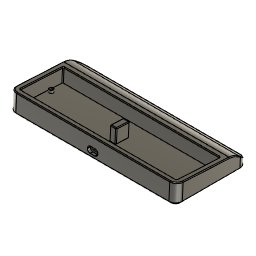
SK-Tsuru (Autodesk Fusion 360 design; units mm, degrees)
Autodesk Fusion 360 part; units mm, degrees
sketch "Base Plane Sketch" plane through (0, 0, 0) normal (0, 0, 1) x (1, 0, 0)
  line L0 (45.9345, 28.7794) -> (255.4845, 28.7794) construction
  line L1 (255.4845, 28.7794) -> (255.4845, 85.9294) construction
  line L2 (255.4845, 85.9294) -> (45.9345, 85.9294) construction
  line L3 (45.9345, 85.9294) -> (45.9345, 28.7794) construction
  line L4 (255.9845, 86.4294) -> (45.4345, 86.4294)
  line L5 (45.4345, 86.4294) -> (45.4345, 28.2794)
  line L6 (45.4345, 28.2794) -> (255.9845, 28.2794)
  line L7 (255.9845, 28.2794) -> (255.9845, 86.4294)
  line L8 (262.8595, 93.3044) -> (38.5595, 93.3044)
  line L9 (38.5595, 93.3044) -> (38.5595, 21.4044)
  line L10 (38.5595, 21.4044) -> (262.8595, 21.4044)
  line L11 (262.8595, 21.4044) -> (262.8595, 93.3044)
  dimension "d180" = 209.55
  dimension "d181" = 57.15
  dimension "d182" = 0.5
  dimension "d183" = 7.375
  constraint horizontal L0
  constraint vertical L1
  constraint horizontal L2
  constraint vertical L3
  measures "d180" distance of L0.start L0.end
  measures "d181" distance of L0.start L2.end
extrude "Extrude19" add sketch "Base Plane Sketch" along normal blind 21.06
extrude "Extrude20" add sketch "Base Plane Sketch" along normal blind 3 contours L4 L5 L6 L7
sketch "Side Plane Sketch" plane through (262.8595, 0, 0) normal (1, 0, 0) x (0, 1, 0)
  line L0 (21.4044, 0) -> (93.3044, 0)
  line L1 (93.3044, 0) -> (93.3044, 21.06)
  line L2 (93.3044, 21.06) -> (21.4044, 21.06)
  line L3 (21.4044, 21.06) -> (21.4044, 0)
  line L4 (93.3044, 21.06) -> (99.8544, 21.06)
  line L5 (99.8544, 21.06) -> (117.0144, 10.0011)
  line L6 (99.8544, 21.06) -> (124.9018, 21.06) construction
  line L7 (93.3044, 0) -> (117.0144, 0)
  line L8 (117.0144, 0) -> (117.0144, 10.0011)
  dimension "d188" = 6.55
  dimension "d189" = 32.8
  dimension "d190" = 23.71
  constraint coincident L1.end L2.start
  constraint perpendicular L1 L4
  constraint horizontal L6
  constraint coincident L0.end L1.start
  constraint perpendicular L1 L7
  constraint perpendicular L7 L8
  measures "d188" distance of L1.end L4.end
  measures "d189" angle of L5 L6
  measures "d190" distance of L0.end L7.end
extrude "Extrude21" add sketch "Side Plane Sketch" against normal up to surface (224.3 mm away) contours L1 L4 L5 L7 L8
sketch "USB C Hole Internal Sketch" plane through (0, 28.2794, 0) normal (0, 1, 0) x (-1, 0, 0)
  line L0 (-255.9845, 3) -> (-45.4345, 3)
  line L1 (-45.4345, 3) -> (-45.4345, 21.06)
  line L2 (-45.4345, 21.06) -> (-255.9845, 21.06)
  line L3 (-255.9845, 21.06) -> (-255.9845, 3)
  line L4 (-255.4845, 21.06) -> (-255.4845, 3) construction
  line L5 (-255.4845, 3) -> (-150.7095, 3) construction
  line L6 (-150.7095, 3) -> (-150.7095, 4.83) construction
  line L7 (-145.9845, 6.66) -> (-155.4345, 6.66)
  line L8 (-155.4345, 6.66) -> (-155.4345, 3)
  line L9 (-155.4345, 3) -> (-145.9845, 3)
  line L10 (-145.9845, 3) -> (-145.9845, 6.66)
  line L11 (-145.9845, 6.66) -> (-155.4345, 3) construction
  line L12 (-155.4345, 6.66) -> (-145.9845, 3) construction
  point P0 (-150.7095, 4.83)
  dimension "d197" = -0.5
  dimension "d198" = 104.775
  dimension "d199" = 1.83
  dimension "d200" = 9.45
  dimension "d201" = 3.66
  constraint perpendicular L4 L5
  constraint perpendicular L5 L6
  constraint horizontal L7
  constraint perpendicular L7 L8
  constraint parallel L7 L9
  constraint parallel L8 L10
  constraint coincident L11 P0
  constraint coincident L12 P0
  constraint coincident P0 L6.end
  measures "d198" distance of L4.end L5.end
  measures "d199" distance of L5.end P0
  measures "d200" distance of L8.end L9.end
  measures "d201" distance of L7.end L8.end
extrude "Extrude22" cut sketch "USB C Hole Internal Sketch" against normal blind 15 contours L0 L7 L8 L9 L10
sketch "USB C Hole External Sketch" plane through (0, 21.4044, 0) normal (0, -1, 0) x (1, 0, 0)
  line L0 (145.9845, 6.66) -> (155.4345, 6.66)
  line L1 (155.4345, 6.66) -> (155.4345, 3)
  line L2 (155.4345, 3) -> (145.9845, 3)
  line L3 (145.9845, 3) -> (145.9845, 6.66)
  line L4 (38.5595, 0) -> (262.8595, 0)
  line L5 (262.8595, 0) -> (262.8595, 21.06)
  line L6 (262.8595, 21.06) -> (38.5595, 21.06)
  line L7 (38.5595, 21.06) -> (38.5595, 0)
  line L8 (145.9845, 3) -> (155.4345, 6.66) construction
  line L9 (155.4345, 3) -> (145.9845, 6.66) construction
  line L10 (157.6845, 8.91) -> (143.7345, 8.91)
  line L11 (143.7345, 8.91) -> (143.7345, 0.75)
  line L12 (143.7345, 0.75) -> (157.6845, 0.75)
  line L13 (157.6845, 0.75) -> (157.6845, 8.91)
  line L14 (157.6845, 8.91) -> (143.7345, 0.75) construction
  line L15 (143.7345, 8.91) -> (157.6845, 0.75) construction
  point P0 (150.7095, 4.83)
  dimension "d204" = 13.95
  dimension "d205" = 8.16
  constraint coincident L2.end L3.start
  constraint coincident L0.end L1.start
  constraint coincident L1.end L2.start
  constraint coincident L0.start L3.end
  constraint horizontal L10
  constraint perpendicular L10 L11
  constraint parallel L10 L12
  constraint parallel L11 L13
  constraint coincident L14 P0
  constraint coincident L15 P0
  constraint midpoint L8 P0
  measures "d204" distance of L11.end L12.end
  measures "d205" distance of L10.end L11.end
extrude "Extrude23" cut sketch "USB C Hole External Sketch" against normal blind 3.875 contours L10 L11 L12 L13
fillet "Fillet8" radius 1.55 4 edges at (145.9845, 26.7794, 3) (145.9845, 26.7794, 6.66) (155.4345, 26.7794, 3) (155.4345, 26.7794, 6.66)
fillet "Fillet9" radius 3.8 4 edges at (143.7345, 23.3419, 8.91) (157.6845, 23.3419, 8.91) (157.6845, 23.3419, 0.75) (143.7345, 23.3419, 0.75)
sketch "Screw Post and Center Blocker Sketch" plane through (0, 0, 3) normal (0, 0, 1) x (-1, 0, 0)
  line L0 (-153.8845, -25.2794) -> (-153.8845, -28.2794)
  line L1 (-153.8845, -28.2794) -> (-255.9845, -28.2794)
  line L2 (-255.9845, -28.2794) -> (-255.9845, -86.4294)
  line L3 (-255.9845, -86.4294) -> (-45.4345, -86.4294)
  line L4 (-45.4345, -86.4294) -> (-45.4345, -28.2794)
  line L5 (-45.4345, -28.2794) -> (-147.5345, -28.2794)
  line L6 (-147.5345, -28.2794) -> (-147.5345, -25.2794)
  line L7 (-147.5345, -25.2794) -> (-153.8845, -25.2794)
  line L8 (-45.9345, -28.7794) -> (-148.0345, -28.7794) construction
  line L9 (-148.0345, -28.7794) -> (-148.0345, -25.7794) construction
  line L10 (-148.0345, -25.7794) -> (-153.3845, -25.7794) construction
  line L11 (-153.3845, -25.7794) -> (-153.3845, -28.7794) construction
  line L12 (-153.3845, -28.7794) -> (-255.4845, -28.7794) construction
  line L13 (-255.4845, -28.7794) -> (-255.4845, -85.9294) construction
  line L14 (-255.4845, -85.9294) -> (-45.9345, -85.9294) construction
  line L15 (-45.9345, -85.9294) -> (-45.9345, -28.7794) construction
  circle A0 centre (-229.2905, -33.8394) radius 2.75
  circle A1 centre (-251.9125, -66.8794) radius 2.75
  circle A2 centre (-72.1285, -33.8394) radius 2.75
  circle A3 centre (-49.5065, -66.8794) radius 2.75
  line L16 (-255.4845, -28.7794) -> (-45.9345, -85.9294) construction
  line L17 (-45.9345, -28.7794) -> (-255.4845, -85.9294) construction
  line L18 (-145.947, -47.8294) -> (-155.472, -47.8294) construction
  line L19 (-155.472, -47.8294) -> (-155.472, -66.8794) construction
  line L20 (-155.472, -66.8794) -> (-145.947, -66.8794) construction
  line L21 (-145.947, -66.8794) -> (-145.947, -47.8294) construction
  line L22 (-145.947, -47.8294) -> (-155.472, -66.8794) construction
  line L23 (-155.472, -47.8294) -> (-145.947, -66.8794) construction
  line L24 (-146.447, -66.3794) -> (-146.447, -48.3294)
  line L25 (-146.447, -48.3294) -> (-154.972, -48.3294)
  line L26 (-154.972, -48.3294) -> (-154.972, -66.3794)
  line L27 (-154.972, -66.3794) -> (-146.447, -66.3794)
  point P0 (-150.7095, -57.3544)
  dimension "d212" = -0.5
  dimension "d213" = 5.5
  dimension "d214" = 5.5
  dimension "d215" = 5.5
  dimension "d216" = 5.5
  dimension "d217" = 26.194
  dimension "d218" = 5.06
  dimension "d219" = 3.572
  dimension "d220" = 19.05
  dimension "d221" = 19.05
  dimension "d222" = 3.572
  dimension "d223" = 26.194
  dimension "d224" = 5.06
  dimension "d225" = 9.525
  dimension "d226" = 19.05
  dimension "d227" = -0.5
  constraint horizontal L18
  constraint perpendicular L18 L19
  constraint parallel L18 L20
  constraint parallel L19 L21
  constraint coincident L22 P0
  constraint coincident L23 P0
  constraint midpoint L16 P0
  measures "d213" diameter of A0
  measures "d214" diameter of A1
  measures "d215" diameter of A2
  measures "d216" diameter of A3
  measures "d217" distance of L13 A0.centre
  measures "d218" distance of L12 A0.centre
  measures "d219" distance of L13 A1.centre
  measures "d220" distance of L14 A1.centre
  measures "d221" distance of L14 A3.centre
  measures "d222" distance of L15 A3.centre
  measures "d223" distance of L15 A2.centre
  measures "d224" distance of L8 A2.centre
  measures "d225" distance of L19.end L20.end
  measures "d226" distance of L18.end L19.end
extrude "Extrude24" add sketch "Screw Post and Center Blocker Sketch" along normal blind 18.06 contours L24 L25 L26 L27
extrude "Extrude25" add sketch "Screw Post and Center Blocker Sketch" along normal blind 3.46 contours A0 | A1 | A2 | A3
hole "Hole9" at (229.2905, 33.8394, 6.46) direction (0, 0, -1) diameter 3.2 depth 4 tip angle 180
hole "Hole10" at (251.9125, 66.8794, 6.46) direction (0, 0, -1) diameter 3.2 depth 4 tip angle 180
hole "Hole11" at (72.1285, 33.8394, 6.46) direction (0, 0, -1) diameter 3.2 depth 4 tip angle 180
hole "Hole12" at (49.5065, 66.8794, 6.46) direction (0, 0, -1) diameter 3.2 depth 4 tip angle 180
fillet "Fillet6" radius 9 4 edges at (262.8595, 117.0144, 5.0006) (262.8595, 21.4044, 10.53) (38.5595, 21.4044, 10.53) (38.5595, 117.0144, 5.0006)
fillet "Fillet7" radius 23.5 1 edges at (150.7095, 99.8544, 21.06)
ref_plane "WorkPlane3" through (150.7095, 117.0144, 0) normal (0, -0.052336, 0.99863) x (-1, 0, 0)
extrude "Extrude26" add 1 faces at (185.0929, 53.2744, 0) along direction (0, 0, -1) up to surface end surface through (150.7095, 117.0144, 0) normal (0, -0.052336, 0.99863) offset 0
fillet "Fillet10" radius 1 8 edges at (255.9845, 28.2794, 12.03) (255.9845, 86.4294, 12.03) (45.4345, 28.2794, 12.03) (154.972, 48.3294, 12.03) (146.447, 48.3294, 12.03) (146.447, 66.3794, 12.03) (154.972, 66.3794, 12.03) (45.4345, 86.4294, 12.03)
chamfer "Chamfer10" distance 1 angle 45 12 edges at (262.8595, 61.6712, 21.06) (262.8595, 99.573, 20.1039) (262.8595, 106.8413, 16.5573) (260.2235, 114.3784, 11.6999) (150.7095, 117.0144, 10.0011) (41.1956, 114.3784, 11.6999) (38.5595, 106.8413, 16.5573) (38.5595, 99.573, 20.1039) (38.5595, 61.6712, 21.06) (41.1956, 24.0405, 21.06) (150.7095, 21.4044, 21.06) (260.2235, 24.0405, 21.06)
chamfer "Chamfer11" distance 3 angle 45 8 edges at (262.8595, 69.2094, -2.5054) (260.2235, 24.0405, -4.8726) (150.7095, 21.4044, -5.0107) (41.1956, 24.0405, -4.8726) (38.5595, 69.2094, -2.5054) (41.1956, 114.3784, -0.1381) (150.7095, 117.0144, 0) (260.2235, 114.3784, -0.1381)
chamfer "Chamfer12" distance 1 angle 45 16 edges at (150.7095, 28.2794, 21.06) (45.7274, 28.5723, 21.06) (45.4345, 57.3544, 21.06) (45.7274, 86.1365, 21.06) (150.7095, 86.4294, 21.06) (255.6916, 86.1365, 21.06) (255.9845, 57.3544, 21.06) (255.6916, 28.5723, 21.06) (146.447, 57.3544, 21.06) (146.7399, 48.6223, 21.06) (150.7095, 48.3294, 21.06) (154.6791, 48.6223, 21.06) (154.972, 57.3544, 21.06) (154.6791, 66.0865, 21.06) (150.7095, 66.3794, 21.06) (146.7399, 66.0865, 21.06)
move_body "Move5" bodies 1 to x (1, 0, 0) y (0, 0.99863, -0.052336) z (0, 0.052336, 0.99863) at (0, 0.1645, 5.9671)
equation "d180 = 19.05 mm * 11"
equation "d181 = 19.05 mm * 3"
equation "d184 = 18.06 mm + 3 mm"
equation "d190 = 17.16 mm + 6.55 mm"
equation "d206 = -4 mm + 0.125 mm"
equation "d221 = d220"
equation "d222 = d219"
equation "d223 = d217"
equation "d224 = d218"
named bodies: "Sk-Tsuru"
